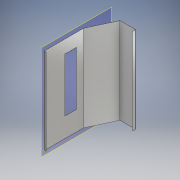
# Autodesk Inventor part: back plate
Saved by Autodesk Inventor 2018 (Build 220112000, 112)
## iProperties
Created: 2018-04-10
Part Number: back plate
Material: Steel
Document SubType Name: Modeling
Designer: P446509
Density: 7.85 g/cm^3
Appearance: Polished Brushed
Author: P446509
Autodesk Inventor part; units mm, degrees
ref_plane "YZ Plane" through (0, 0, 0) normal (1, 0, 0) x (0, 1, 0)
ref_plane "XZ Plane" through (0, 0, 0) normal (0, 1, 0) x (-1, 0, 0)
ref_plane "XY Plane" through (0, 0, 0) normal (0, 0, 1) x (1, 0, 0)
sketch "Sketch1" plane through (0, 0, 0) normal (0, 0, 1) x (1, 0, 0)
  line L0 (20, 0) -> (0, 0)
  line L1 (0, 0) -> (0, 500)
  line L2 (0, 500) -> (147.9164, 817.2077)
  line L3 (147.9164, 817.2077) -> (347.9164, 817.2077)
  line L4 (347.9164, 817.2077) -> (347.9164, 777.2077)
  line L5 (346.3164, 777.2077) -> (346.3164, 815.6077)
  line L6 (346.3164, 815.6077) -> (148.9357, 815.6077)
  line L7 (148.9357, 815.6077) -> (1.6, 499.6453)
  line L8 (1.6, 499.6453) -> (1.6, 1.6)
  line L9 (1.6, 1.6) -> (20, 1.6)
  line L10 (20, 1.6) -> (20, 0)
  line L11 (346.3164, 777.2077) -> (347.9164, 777.2077)
  dimension "d0" = 155
  dimension "d1" = 500
  dimension "d2" = 350
  dimension "d3" = 200
  dimension "d4" = 20
  dimension "d5" = 40
  dimension "d6" = 1.6
  constraints: 24 end point, 4 perpendicular, 2 parallel, 1 horizontal, 1 vertical, 4 other
  measures "d0" angle of L2 L1
  measures "d1" distance of L0.end L1.end
  measures "d2" distance of L1.end L2.end
  measures "d3" distance of L2.end L3.end
  measures "d4" distance of L0.start L0.end
  measures "d5" distance of L3.end L4.end
  measures "d6" distance between parallel lines of L1 L8
extrude "main" add sketch "Sketch1" along normal blind 1100
ref_plane "Work Plane1" through (0.8, 0, 0) normal (-1, 0, 0) x (0, 0, 1)
sketch "Sketch4" plane through (0.8, 0, 0) normal (-1, 0, 0) x (0, 0, 1)
  point P0 (0, 0)
sketch "Sketch6" plane through (0, 0, 0) normal (-1, 0, 0) x (0, 0, 1)
  line L0 (0, 0) -> (1100, 0) projected
  line L1 (1100, 0) -> (674.534, 0)
  line L2 (934.534, 410.312) -> (249.534, 410.312)
  line L3 (249.534, 410.312) -> (249.534, 260.312)
  line L4 (249.534, 260.312) -> (934.534, 260.312)
  line L5 (934.534, 260.312) -> (934.534, 410.312)
  line L6 (0, 1.6) -> (1100, 1.6) projected
  dimension "d27" = 685
  dimension "d28" = 258.712
  constraints: 10 end point, 2 horizontal, 2 parallel, 1 perpendicular
  measures "d27" distance of L4.end L3.end
  measures "d28" distance between parallel lines of L4 L6
extrude "Extrusion4" cut sketch "Sketch6" against normal blind 25.5
body "Solid1"
